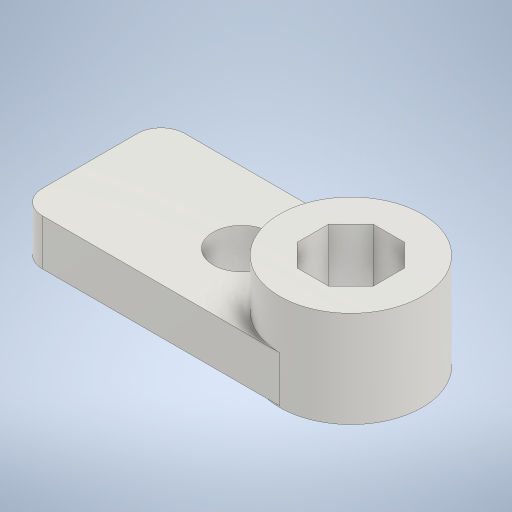
# Autodesk Inventor part: Bauteil1
Saved by Autodesk Inventor 2024.3 (Build 283343000, 343)
## iProperties
Created: 2025-08-22
Part Number: Bauteil1
Material: 1.0038 S235JR
Document SubType Name: Modeling
Designer: Dickert.Jonas
Density: 7.86 g/cm^3
Appearance: Stahl
Author: Dickert.Jonas
Autodesk Inventor part; units mm, degrees
ref_plane "YZ Plane" through (0, 0, 0) normal (1, 0, 0) x (0, 1, 0)
ref_plane "XZ Plane" through (0, 0, 0) normal (0, 1, 0) x (-1, 0, 0)
ref_plane "XY Plane" through (0, 0, 0) normal (0, 0, 1) x (1, 0, 0)
sketch "Skizze1" plane through (0, 0, 0) normal (0, 0, 1) x (1, 0, 0)
  line L0 (0, -21) -> (0, 21) projected
  line L1 (-35, -15) -> (20, -15)
  line L2 (20, 15) -> (-35, 15)
  line L3 (-35, 15) -> (-35, -15)
  line L4 (20, 15) -> (9.0192, 15)
  line L5 (9.0192, -15) -> (20, -15)
  circle A0 centre (20, 0) radius 15
  line L6 (23.3137, 8) -> (28, 3.3137)
  line L7 (28, 3.3137) -> (28, -3.3137)
  line L8 (28, -3.3137) -> (23.3137, -8)
  line L9 (23.3137, -8) -> (16.6863, -8)
  line L10 (16.6863, -8) -> (12, -3.3137)
  line L11 (12, -3.3137) -> (12, 3.3137)
  line L12 (12, 3.3137) -> (16.6863, 8)
  line L13 (16.6863, 8) -> (23.3137, 8)
  line L14 (-49, 0) -> (49, 0) projected
  point P0 (0, 0)
  point P1 (20, -15)
  point P2 (20, 15)
  point P3 (-3, 0)
  dimension "d18" = 16
  constraints: 26 end point, 2 horizontal, 2 parallel, 2 point on circle, 1 centre point, 1 coincident, 1 point on line, 17 other
  measures "d18" distance between parallel lines of L9 L13
extrude "Extrusion1" add sketch "Skizze1" against normal blind 9.7
extrude "Extrusion2" add sketch "Skizze1" against normal blind 10 contours L14 L11 L10 L9 L8 L7 A0 | A0 L14 L7 L6 L13 L12 L11 | L14 L7 L8 L9 L10 L11 | L11 L12 L13 L6 L7 L14
fillet "Rundung1" radius 5 2 edges at (-35, -15, -4.85) (-35, 15, -4.85)
hole "Bohrung1" at (-3, 0, 0) direction (0, 0, -1) diameter 12 end through all
extrude "Extrusion3" add sketch "Skizze1" along normal blind 10.3 contours L14 L11 L10 L9 L8 L7 A0 | A0 L14 L7 L6 L13 L12 L11 | L14 L7 L8 L9 L10 L11 | L11 L12 L13 L6 L7 L14
extrude "Extrusion4" cut sketch "Skizze1" along normal blind 10.3 contours L14 L7 L8 L9 L10 L11 | L11 L12 L13 L6 L7 L14
extrude "Extrusion5" cut sketch "Skizze1" against normal blind 10 contours L14 L7 L8 L9 L10 L11 | L11 L12 L13 L6 L7 L14
